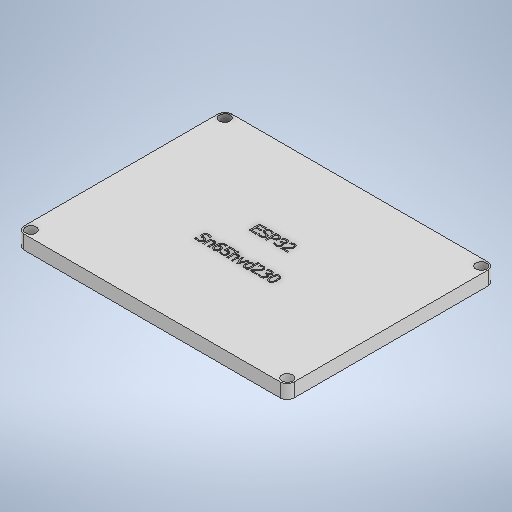
# Autodesk Inventor part: esp_can_case_lid
Saved by Autodesk Inventor 2025 (Build 290162000, 162)
## iProperties
Created: 2025-01-20
Part Number: esp_can_case_lid
Material: Generic
Document SubType Name: Modeling
Designer: danielrachi
Density: 1 g/cm^3
Appearance: Default
Author: danielrachi
Autodesk Inventor part; units mm, degrees
ref_plane "YZ Plane" through (0, 0, 0) normal (1, 0, 0) x (0, 1, 0)
ref_plane "XZ Plane" through (0, 0, 0) normal (0, 1, 0) x (-1, 0, 0)
ref_plane "XY Plane" through (0, 0, 0) normal (0, 0, 1) x (1, 0, 0)
sketch "Sketch1" plane through (0, 0, 0) normal (0, 1, 0) x (-1, 0, 0)
  line L0 (-39, 30) -> (39, 30)
  line L1 (39, 30) -> (39, -30)
  line L2 (39, -30) -> (-39, -30)
  line L3 (-39, -30) -> (-39, 30)
  line L4 (-39, 30) -> (39, -30) construction
  line L5 (39, 30) -> (-39, -30) construction
  point P0 (0, 0)
  dimension "d0" = 78
  dimension "d1" = 60
  constraints: 12 end point, 2 midpoint, 2 parallel, 1 horizontal, 1 perpendicular
  measures "d0" distance of L1.end L2.end
  measures "d1" distance of L0.end L1.end
extrude "Extrusion1" add sketch "Sketch1" along normal blind 4
sketch "Sketch2" plane through (0, 4, 0) normal (0, 1, 0) x (1, 0, 0)
  circle A0 centre (37, -28) radius 1.55
  line L0 (-39, -30) -> (39, -30) projected
  line L1 (39, -30) -> (39, 30) projected
  line L2 (-39, 30) -> (-39, -30) projected
  line L3 (-39, 0) -> (39, 0)
  line L4 (39, 30) -> (-39, 30) projected
  line L5 (0, 30) -> (0, -30)
  circle A1 centre (-37, -28) radius 1.55
  circle A2 centre (37, 28) radius 1.55
  circle A3 centre (-37, 28) radius 1.55
  line L6 (-39, 30) -> (39, 30) construction
  line L7 (39, 30) -> (39, -30) construction
  line L8 (39, -30) -> (-39, -30) construction
  line L9 (-39, -30) -> (-39, 30) construction
  line L10 (-5.4773, 3.4945) -> (-5.4773, 6.5425)
  line L11 (-5.4773, 6.5425) -> (-3.5704, 6.5425)
  line L12 (-3.5704, 6.5425) -> (-3.5704, 6.1818)
  line L13 (-3.5704, 6.1818) -> (-5.0722, 6.1818)
  line L14 (-5.0722, 6.1818) -> (-5.0722, 5.347)
  line L15 (-5.0722, 5.347) -> (-3.6717, 5.347)
  line L16 (-3.6717, 5.347) -> (-3.6717, 4.9863)
  line L17 (-3.6717, 4.9863) -> (-5.0722, 4.9863)
  line L18 (-5.0722, 4.9863) -> (-5.0722, 3.8551)
  line L19 (-5.0722, 3.8551) -> (-3.5704, 3.8551)
  line L20 (-3.5704, 3.8551) -> (-3.5704, 3.4945)
  line L21 (-3.5704, 3.4945) -> (-5.4773, 3.4945)
  spline S0 degree 2 poles (-2.2761, 3.4401) (-2.6071, 3.4401) (-3.0715, 3.5784) (-3.2765, 3.6772) knots 0 0 0 1 2 2 2
  line L22 (-3.2765, 3.6772) -> (-3.2765, 4.1861)
  line L23 (-3.2765, 4.1861) -> (-3.2468, 4.1861)
  spline S1 degree 2 poles (-3.2468, 4.1861) (-3.0468, 3.9983) (-2.5404, 3.7909) (-2.3058, 3.7909) knots 0 0 0 1 2 2 2
  spline S2 degree 2 poles (-2.3058, 3.7909) (-1.9698, 3.7909) (-1.6265, 4.07) (-1.6265, 4.2997) knots 0 0 0 1 2 2 2
  spline S3 degree 2 poles (-1.6265, 4.2997) (-1.6265, 4.4825) (-1.8068, 4.7097) (-2.0019, 4.7665) knots 0 0 0 1 2 2 2
  spline S4 degree 2 poles (-2.0019, 4.7665) (-2.1427, 4.806) (-2.3774, 4.8604) (-2.5528, 4.9048) knots 0 0 0 1 2 2 2
  spline S5 degree 2 poles (-2.5528, 4.9048) (-2.7108, 4.9468) (-2.9603, 5.0728) (-3.0566, 5.1741) knots 0 0 0 1 2 2 2
  spline S6 degree 2 poles (-3.0566, 5.1741) (-3.1505, 5.2753) (-3.2542, 5.547) (-3.2542, 5.7249) knots 0 0 0 1 2 2 2
  spline S7 degree 2 poles (-3.2542, 5.7249) (-3.2542, 6.0954) (-2.6763, 6.5968) (-2.2292, 6.5968) knots 0 0 0 1 2 2 2
  spline S8 degree 2 poles (-2.2292, 6.5968) (-1.9723, 6.5968) (-1.5178, 6.4955) (-1.3227, 6.3992) knots 0 0 0 1 2 2 2
  line L24 (-1.3227, 6.3992) -> (-1.3227, 5.9151)
  line L25 (-1.3227, 5.9151) -> (-1.3523, 5.9151)
  spline S9 degree 2 poles (-1.3523, 5.9151) (-1.4981, 6.0484) (-1.9525, 6.246) (-2.202, 6.246) knots 0 0 0 1 2 2 2
  spline S10 degree 2 poles (-2.202, 6.246) (-2.4836, 6.246) (-2.8319, 5.9818) (-2.8319, 5.7669) knots 0 0 0 1 2 2 2
  spline S11 degree 2 poles (-2.8319, 5.7669) (-2.8319, 5.5742) (-2.6269, 5.3445) (-2.4342, 5.2926) knots 0 0 0 1 2 2 2
  spline S12 degree 2 poles (-2.4342, 5.2926) (-2.3058, 5.258) (-1.9328, 5.1691) (-1.8093, 5.1321) knots 0 0 0 1 2 2 2
  spline S13 degree 2 poles (-1.8093, 5.1321) (-1.4956, 5.0357) (-1.2041, 4.6479) (-1.2041, 4.3639) knots 0 0 0 1 2 2 2
  spline S14 degree 2 poles (-1.2041, 4.3639) (-1.2041, 4.1836) (-1.3499, 3.8378) (-1.4808, 3.7168) knots 0 0 0 1 2 2 2
  spline S15 degree 2 poles (-1.4808, 3.7168) (-1.6265, 3.5834) (-1.997, 3.4401) (-2.2761, 3.4401) knots 0 0 0 1 2 2 2
  spline S16 degree 2 poles (1.135, 5.6236) (1.135, 5.426) (0.9942, 5.0703) (0.8682, 4.9468) knots 0 0 0 1 2 2 2
  spline S17 degree 2 poles (0.8682, 4.9468) (0.7101, 4.7912) (0.2828, 4.6307) (-0.0432, 4.6307) knots 0 0 0 1 2 2 2
  line L26 (-0.0432, 4.6307) -> (-0.3866, 4.6307)
  line L27 (-0.3866, 4.6307) -> (-0.3866, 3.4945)
  line L28 (-0.3866, 3.4945) -> (-0.7916, 3.4945)
  line L29 (-0.7916, 3.4945) -> (-0.7916, 6.5425)
  line L30 (-0.7916, 6.5425) -> (-0.0259, 6.5425)
  spline S18 degree 2 poles (-0.0259, 6.5425) (0.2458, 6.5425) (0.6261, 6.4535) (0.7719, 6.3523) knots 0 0 0 1 2 2 2
  spline S19 degree 2 poles (0.7719, 6.3523) (0.9423, 6.2362) (1.135, 5.878) (1.135, 5.6236) knots 0 0 0 1 2 2 2
  spline S20 degree 2 poles (0.7126, 5.6113) (0.7126, 5.7693) (0.6039, 6.0015) (0.4928, 6.0756) knots 0 0 0 1 2 2 2
  spline S21 degree 2 poles (0.4928, 6.0756) (0.3964, 6.1398) (0.1396, 6.1917) (-0.0506, 6.1917) knots 0 0 0 1 2 2 2
  line L31 (-0.0506, 6.1917) -> (-0.3866, 6.1917)
  line L32 (-0.3866, 6.1917) -> (-0.3866, 4.9765)
  line L33 (-0.3866, 4.9765) -> (-0.1099, 4.9765)
  spline S22 degree 2 poles (-0.1099, 4.9765) (0.1371, 4.9765) (0.4409, 5.0555) (0.5397, 5.1592) knots 0 0 0 1 2 2 2
  spline S23 degree 2 poles (0.5397, 5.1592) (0.6311, 5.2506) (0.7126, 5.4655) (0.7126, 5.6113) knots 0 0 0 1 2 2 2
  spline S24 degree 2 poles (2.2564, 6.2535) (2.1452, 6.2535) (1.9254, 6.1991) (1.8192, 6.1571) knots 0 0 0 1 2 2 2
  spline S25 degree 2 poles (1.8192, 6.1571) (1.7204, 6.1151) (1.5746, 6.0262) (1.5178, 5.9867) knots 0 0 0 1 2 2 2
  line L34 (1.5178, 5.9867) -> (1.4931, 5.9867)
  line L35 (1.4931, 5.9867) -> (1.4931, 6.419)
  spline S26 degree 2 poles (1.4931, 6.419) (1.6265, 6.4906) (2.0835, 6.6067) (2.2885, 6.6067) knots 0 0 0 1 2 2 2
  spline S27 degree 2 poles (2.2885, 6.6067) (2.496, 6.6067) (2.8047, 6.5227) (2.9307, 6.4338) knots 0 0 0 1 2 2 2
  spline S28 degree 2 poles (2.9307, 6.4338) (3.0641, 6.3374) (3.2024, 6.0583) (3.2024, 5.8706) knots 0 0 0 1 2 2 2
  spline S29 degree 2 poles (3.2024, 5.8706) (3.2024, 5.6187) (2.8714, 5.2383) (2.6392, 5.1889) knots 0 0 0 1 2 2 2
  line L36 (2.6392, 5.1889) -> (2.6392, 5.1592)
  spline S30 degree 2 poles (2.6392, 5.1592) (2.7355, 5.1395) (2.9554, 5.0506) (3.0492, 4.9616) knots 0 0 0 1 2 2 2
  spline S31 degree 2 poles (3.0492, 4.9616) (3.1431, 4.8752) (3.2617, 4.5985) (3.2617, 4.3985) knots 0 0 0 1 2 2 2
  spline S32 degree 2 poles (3.2617, 4.3985) (3.2617, 4.1935) (3.1209, 3.8452) (2.9924, 3.7118) knots 0 0 0 1 2 2 2
  spline S33 degree 2 poles (2.9924, 3.7118) (2.859, 3.5735) (2.4811, 3.4302) (2.2415, 3.4302) knots 0 0 0 1 2 2 2
  spline S34 degree 2 poles (2.2415, 3.4302) (2.0118, 3.4302) (1.5623, 3.5414) (1.4091, 3.618) knots 0 0 0 1 2 2 2
  line L37 (1.4091, 3.618) -> (1.4091, 4.0502)
  line L38 (1.4091, 4.0502) -> (1.4388, 4.0502)
  spline S35 degree 2 poles (1.4388, 4.0502) (1.5672, 3.9563) (2.0019, 3.7834) (2.2168, 3.7834) knots 0 0 0 1 2 2 2
  spline S36 degree 2 poles (2.2168, 3.7834) (2.3428, 3.7834) (2.5948, 3.8625) (2.6787, 3.9539) knots 0 0 0 1 2 2 2
  spline S37 degree 2 poles (2.6787, 3.9539) (2.7602, 4.0453) (2.8467, 4.2626) (2.8467, 4.4281) knots 0 0 0 1 2 2 2
  spline S38 degree 2 poles (2.8467, 4.4281) (2.8467, 4.5936) (2.7504, 4.8085) (2.6639, 4.8703) knots 0 0 0 1 2 2 2
  spline S39 degree 2 poles (2.6639, 4.8703) (2.5775, 4.932) (2.3428, 4.9789) (2.2045, 4.9789) knots 0 0 0 1 2 2 2
  line L39 (2.2045, 4.9789) -> (2.0316, 4.9789)
  line L40 (2.0316, 4.9789) -> (2.0316, 5.3173)
  line L41 (2.0316, 5.3173) -> (2.1674, 5.3173)
  spline S40 degree 2 poles (2.1674, 5.3173) (2.4416, 5.3173) (2.7874, 5.5791) (2.7874, 5.8286) knots 0 0 0 1 2 2 2
  spline S41 degree 2 poles (2.7874, 5.8286) (2.7874, 5.9447) (2.6985, 6.1102) (2.6269, 6.1596) knots 0 0 0 1 2 2 2
  spline S42 degree 2 poles (2.6269, 6.1596) (2.5503, 6.2115) (2.3626, 6.2535) (2.2564, 6.2535) knots 0 0 0 1 2 2 2
  line L42 (5.6008, 3.4945) -> (3.7211, 3.4945)
  line L43 (3.7211, 3.4945) -> (3.7211, 3.9267)
  spline S43 degree 2 poles (3.7211, 3.9267) (3.9236, 4.1169) (4.2842, 4.4701) (4.4571, 4.6603) knots 0 0 0 1 2 2 2
  spline S44 degree 2 poles (4.4571, 4.6603) (4.8054, 5.0432) (5.0598, 5.5026) (5.0598, 5.7471) knots 0 0 0 1 2 2 2
  spline S45 degree 2 poles (5.0598, 5.7471) (5.0598, 5.8755) (4.9808, 6.0682) (4.9092, 6.13) knots 0 0 0 1 2 2 2
  spline S46 degree 2 poles (4.9092, 6.13) (4.8375, 6.1917) (4.6498, 6.2535) (4.5362, 6.2535) knots 0 0 0 1 2 2 2
  spline S47 degree 2 poles (4.5362, 6.2535) (4.4275, 6.2535) (4.2052, 6.1991) (4.1039, 6.1571) knots 0 0 0 1 2 2 2
  spline S48 degree 2 poles (4.1039, 6.1571) (4.0175, 6.1225) (3.8569, 6.0237) (3.8075, 5.9892) knots 0 0 0 1 2 2 2
  line L44 (3.8075, 5.9892) -> (3.7853, 5.9892)
  line L45 (3.7853, 5.9892) -> (3.7853, 6.4239)
  spline S49 degree 2 poles (3.7853, 6.4239) (3.9113, 6.4856) (4.3633, 6.6067) (4.5658, 6.6067) knots 0 0 0 1 2 2 2
  spline S50 degree 2 poles (4.5658, 6.6067) (4.9931, 6.6067) (5.4748, 6.1547) (5.4748, 5.7693) knots 0 0 0 1 2 2 2
  spline S51 degree 2 poles (5.4748, 5.7693) (5.4748, 5.589) (5.3908, 5.2877) (5.3167, 5.1592) knots 0 0 0 1 2 2 2
  spline S52 degree 2 poles (5.3167, 5.1592) (5.2426, 5.0259) (5.0277, 4.764) (4.9092, 4.6381) knots 0 0 0 1 2 2 2
  spline S53 degree 2 poles (4.9092, 4.6381) (4.7165, 4.4281) (4.2447, 3.9786) (4.1039, 3.8477) knots 0 0 0 1 2 2 2
  line L46 (4.1039, 3.8477) -> (5.6008, 3.8477)
  line L47 (5.6008, 3.8477) -> (5.6008, 3.4945)
  spline S54 degree 2 poles (-10.2654, -6.5968) (-10.5964, -6.5968) (-11.0607, -6.4585) (-11.2657, -6.3597) knots 0 0 0 1 2 2 2
  line L48 (-11.2657, -6.3597) -> (-11.2657, -5.8508)
  line L49 (-11.2657, -5.8508) -> (-11.2361, -5.8508)
  spline S55 degree 2 poles (-11.2361, -5.8508) (-11.036, -6.0386) (-10.5297, -6.246) (-10.295, -6.246) knots 0 0 0 1 2 2 2
  spline S56 degree 2 poles (-10.295, -6.246) (-9.9591, -6.246) (-9.6158, -5.9669) (-9.6158, -5.7372) knots 0 0 0 1 2 2 2
  spline S57 degree 2 poles (-9.6158, -5.7372) (-9.6158, -5.5544) (-9.7961, -5.3272) (-9.9912, -5.2704) knots 0 0 0 1 2 2 2
  spline S58 degree 2 poles (-9.9912, -5.2704) (-10.132, -5.2309) (-10.3667, -5.1765) (-10.542, -5.1321) knots 0 0 0 1 2 2 2
  spline S59 degree 2 poles (-10.542, -5.1321) (-10.7001, -5.0901) (-10.9496, -4.9641) (-11.0459, -4.8628) knots 0 0 0 1 2 2 2
  spline S60 degree 2 poles (-11.0459, -4.8628) (-11.1398, -4.7616) (-11.2435, -4.4899) (-11.2435, -4.312) knots 0 0 0 1 2 2 2
  spline S61 degree 2 poles (-11.2435, -4.312) (-11.2435, -3.9415) (-10.6655, -3.4401) (-10.2185, -3.4401) knots 0 0 0 1 2 2 2
  spline S62 degree 2 poles (-10.2185, -3.4401) (-9.9616, -3.4401) (-9.5071, -3.5414) (-9.312, -3.6377) knots 0 0 0 1 2 2 2
  line L50 (-9.312, -3.6377) -> (-9.312, -4.1218)
  line L51 (-9.312, -4.1218) -> (-9.3416, -4.1218)
  spline S63 degree 2 poles (-9.3416, -4.1218) (-9.4873, -3.9885) (-9.9418, -3.7909) (-10.1913, -3.7909) knots 0 0 0 1 2 2 2
  spline S64 degree 2 poles (-10.1913, -3.7909) (-10.4729, -3.7909) (-10.8211, -4.0551) (-10.8211, -4.27) knots 0 0 0 1 2 2 2
  spline S65 degree 2 poles (-10.8211, -4.27) (-10.8211, -4.4627) (-10.6161, -4.6924) (-10.4235, -4.7443) knots 0 0 0 1 2 2 2
  spline S66 degree 2 poles (-10.4235, -4.7443) (-10.295, -4.7789) (-9.9221, -4.8678) (-9.7986, -4.9048) knots 0 0 0 1 2 2 2
  spline S67 degree 2 poles (-9.7986, -4.9048) (-9.4849, -5.0012) (-9.1934, -5.389) (-9.1934, -5.673) knots 0 0 0 1 2 2 2
  spline S68 degree 2 poles (-9.1934, -5.673) (-9.1934, -5.8533) (-9.3391, -6.1991) (-9.47, -6.3202) knots 0 0 0 1 2 2 2
  spline S69 degree 2 poles (-9.47, -6.3202) (-9.6158, -6.4535) (-9.9863, -6.5968) (-10.2654, -6.5968) knots 0 0 0 1 2 2 2
  line L52 (-7.0148, -6.5425) -> (-7.4002, -6.5425)
  line L53 (-7.4002, -6.5425) -> (-7.4002, -5.2383)
  spline S70 degree 2 poles (-7.4002, -5.2383) (-7.4002, -5.0802) (-7.4298, -4.8085) (-7.4743, -4.727) knots 0 0 0 1 2 2 2
  spline S71 degree 2 poles (-7.4743, -4.727) (-7.5212, -4.6405) (-7.6892, -4.5566) (-7.8324, -4.5566) knots 0 0 0 1 2 2 2
  spline S72 degree 2 poles (-7.8324, -4.5566) (-7.9757, -4.5566) (-8.2795, -4.7097) (-8.4252, -4.8332) knots 0 0 0 1 2 2 2
  line L54 (-8.4252, -4.8332) -> (-8.4252, -6.5425)
  line L55 (-8.4252, -6.5425) -> (-8.8105, -6.5425)
  line L56 (-8.8105, -6.5425) -> (-8.8105, -4.2552)
  line L57 (-8.8105, -4.2552) -> (-8.4252, -4.2552)
  line L58 (-8.4252, -4.2552) -> (-8.4252, -4.5096)
  spline S73 degree 2 poles (-8.4252, -4.5096) (-8.2523, -4.354) (-7.9189, -4.191) (-7.7312, -4.191) knots 0 0 0 1 2 2 2
  spline S74 degree 2 poles (-7.7312, -4.191) (-7.3952, -4.191) (-7.0148, -4.6356) (-7.0148, -5.058) knots 0 0 0 1 2 2 2
  line L59 (-7.0148, -5.058) -> (-7.0148, -6.5425)
  spline S75 degree 2 poles (-4.6041, -5.5544) (-4.6041, -5.7891) (-4.7597, -6.1868) (-4.8906, -6.3202) knots 0 0 0 1 2 2 2
  spline S76 degree 2 poles (-4.8906, -6.3202) (-5.0265, -6.4609) (-5.3673, -6.6067) (-5.5724, -6.6067) knots 0 0 0 1 2 2 2
  spline S77 degree 2 poles (-5.5724, -6.6067) (-5.7774, -6.6067) (-6.1158, -6.4684) (-6.2442, -6.33) knots 0 0 0 1 2 2 2
  spline S78 degree 2 poles (-6.2442, -6.33) (-6.4023, -6.1645) (-6.5801, -5.6088) (-6.5801, -5.2037) knots 0 0 0 1 2 2 2
  spline S79 degree 2 poles (-6.5801, -5.2037) (-6.5801, -4.806) (-6.4171, -4.1663) (-6.2467, -3.9292) knots 0 0 0 1 2 2 2
  spline S80 degree 2 poles (-6.2467, -3.9292) (-6.0812, -3.697) (-5.5575, -3.4376) (-5.2142, -3.4376) knots 0 0 0 1 2 2 2
  spline S81 degree 2 poles (-5.2142, -3.4376) (-5.1129, -3.4376) (-4.9351, -3.4574) (-4.8684, -3.4796) knots 0 0 0 1 2 2 2
  line L60 (-4.8684, -3.4796) -> (-4.8684, -3.8724)
  line L61 (-4.8684, -3.8724) -> (-4.8857, -3.8724)
  spline S82 degree 2 poles (-4.8857, -3.8724) (-4.9425, -3.8427) (-5.15, -3.7909) (-5.2685, -3.7909) knots 0 0 0 1 2 2 2
  spline S83 degree 2 poles (-5.2685, -3.7909) (-5.6489, -3.7909) (-6.1158, -4.3046) (-6.1602, -4.8085) knots 0 0 0 1 2 2 2
  spline S84 degree 2 poles (-6.1602, -4.8085) (-6.0145, -4.7072) (-5.7082, -4.5961) (-5.5254, -4.5961) knots 0 0 0 1 2 2 2
  spline S85 degree 2 poles (-5.5254, -4.5961) (-5.3476, -4.5961) (-5.0808, -4.6677) (-4.9351, -4.7764) knots 0 0 0 1 2 2 2
  spline S86 degree 2 poles (-4.9351, -4.7764) (-4.7671, -4.9024) (-4.6041, -5.2926) (-4.6041, -5.5544) knots 0 0 0 1 2 2 2
  spline S87 degree 2 poles (-5.0191, -5.5717) (-5.0191, -5.384) (-5.1179, -5.1296) (-5.2266, -5.0407) knots 0 0 0 1 2 2 2
  spline S88 degree 2 poles (-5.2266, -5.0407) (-5.3081, -4.9765) (-5.5106, -4.9345) (-5.6168, -4.9345) knots 0 0 0 1 2 2 2
  spline S89 degree 2 poles (-5.6168, -4.9345) (-5.7601, -4.9345) (-6.0293, -5.0209) (-6.1602, -5.1024) knots 0 0 0 1 2 2 2
  spline S90 degree 2 poles (-6.1602, -5.1024) (-6.1627, -5.1469) (-6.1676, -5.2309) (-6.1676, -5.2951) knots 0 0 0 1 2 2 2
  spline S91 degree 2 poles (-6.1676, -5.2951) (-6.1676, -5.6113) (-6.0441, -5.999) (-5.9503, -6.1003) knots 0 0 0 1 2 2 2
  spline S92 degree 2 poles (-5.9503, -6.1003) (-5.8638, -6.1966) (-5.6761, -6.2732) (-5.5699, -6.2732) knots 0 0 0 1 2 2 2
  spline S93 degree 2 poles (-5.5699, -6.2732) (-5.3229, -6.2732) (-5.0191, -5.9225) (-5.0191, -5.5717) knots 0 0 0 1 2 2 2
  spline S94 degree 2 poles (-2.3959, -5.5742) (-2.3959, -5.794) (-2.5367, -6.1695) (-2.6651, -6.3078) knots 0 0 0 1 2 2 2
  spline S95 degree 2 poles (-2.6651, -6.3078) (-2.7936, -6.4461) (-3.1764, -6.6067) (-3.4136, -6.6067) knots 0 0 0 1 2 2 2
  spline S96 degree 2 poles (-3.4136, -6.6067) (-3.6309, -6.6067) (-4.0558, -6.5103) (-4.2114, -6.4338) knots 0 0 0 1 2 2 2
  line L62 (-4.2114, -6.4338) -> (-4.2114, -6.0015)
  line L63 (-4.2114, -6.0015) -> (-4.1817, -6.0015)
  spline S97 degree 2 poles (-4.1817, -6.0015) (-4.1348, -6.0361) (-3.9594, -6.125) (-3.8532, -6.1645) knots 0 0 0 1 2 2 2
  spline S98 degree 2 poles (-3.8532, -6.1645) (-3.7322, -6.2065) (-3.5321, -6.2535) (-3.4062, -6.2535) knots 0 0 0 1 2 2 2
  spline S99 degree 2 poles (-3.4062, -6.2535) (-3.2827, -6.2535) (-3.0505, -6.1645) (-2.9665, -6.0682) knots 0 0 0 1 2 2 2
  spline S100 degree 2 poles (-2.9665, -6.0682) (-2.8899, -5.9768) (-2.8109, -5.7348) (-2.8109, -5.5717) knots 0 0 0 1 2 2 2
  spline S101 degree 2 poles (-2.8109, -5.5717) (-2.8109, -5.4087) (-2.8998, -5.2012) (-2.9838, -5.1321) knots 0 0 0 1 2 2 2
  spline S102 degree 2 poles (-2.9838, -5.1321) (-3.0702, -5.0555) (-3.3271, -4.9913) (-3.4827, -4.9913) knots 0 0 0 1 2 2 2
  spline S103 degree 2 poles (-3.4827, -4.9913) (-3.6507, -4.9913) (-3.9841, -5.0432) (-4.0854, -5.0654) knots 0 0 0 1 2 2 2
  line L64 (-4.0854, -5.0654) -> (-4.0854, -3.4945)
  line L65 (-4.0854, -3.4945) -> (-2.4132, -3.4945)
  line L66 (-2.4132, -3.4945) -> (-2.4132, -3.8526)
  line L67 (-2.4132, -3.8526) -> (-3.6927, -3.8526)
  line L68 (-3.6927, -3.8526) -> (-3.6927, -4.6652)
  spline S104 degree 2 poles (-3.6927, -4.6652) (-3.6186, -4.6554) (-3.4753, -4.6479) (-3.416, -4.6479) knots 0 0 0 1 2 2 2
  spline S105 degree 2 poles (-3.416, -4.6479) (-3.1814, -4.6479) (-2.8578, -4.7245) (-2.7096, -4.8381) knots 0 0 0 1 2 2 2
  spline S106 degree 2 poles (-2.7096, -4.8381) (-2.5589, -4.9518) (-2.3959, -5.2976) (-2.3959, -5.5742) knots 0 0 0 1 2 2 2
  line L69 (-0.1037, -6.5425) -> (-0.4891, -6.5425)
  line L70 (-0.4891, -6.5425) -> (-0.4891, -5.2383)
  spline S107 degree 2 poles (-0.4891, -5.2383) (-0.4891, -5.0802) (-0.5187, -4.8085) (-0.5632, -4.727) knots 0 0 0 1 2 2 2
  spline S108 degree 2 poles (-0.5632, -4.727) (-0.6101, -4.6405) (-0.7781, -4.5566) (-0.9213, -4.5566) knots 0 0 0 1 2 2 2
  spline S109 degree 2 poles (-0.9213, -4.5566) (-1.0646, -4.5566) (-1.3684, -4.7097) (-1.5141, -4.8332) knots 0 0 0 1 2 2 2
  line L71 (-1.5141, -4.8332) -> (-1.5141, -6.5425)
  line L72 (-1.5141, -6.5425) -> (-1.8994, -6.5425)
  line L73 (-1.8994, -6.5425) -> (-1.8994, -3.3586)
  line L74 (-1.8994, -3.3586) -> (-1.5141, -3.3586)
  line L75 (-1.5141, -3.3586) -> (-1.5141, -4.5096)
  spline S110 degree 2 poles (-1.5141, -4.5096) (-1.3412, -4.354) (-1.0078, -4.191) (-0.82, -4.191) knots 0 0 0 1 2 2 2
  spline S111 degree 2 poles (-0.82, -4.191) (-0.4841, -4.191) (-0.1037, -4.6356) (-0.1037, -5.058) knots 0 0 0 1 2 2 2
  line L76 (-0.1037, -5.058) -> (-0.1037, -6.5425)
  line L77 (2.2329, -4.2552) -> (1.3709, -6.5425)
  line L78 (1.3709, -6.5425) -> (1.0251, -6.5425)
  line L79 (1.0251, -6.5425) -> (0.1704, -4.2552)
  line L80 (0.1704, -4.2552) -> (0.5879, -4.2552)
  line L81 (0.5879, -4.2552) -> (1.2128, -6.0163)
  line L82 (1.2128, -6.0163) -> (1.8328, -4.2552)
  line L83 (1.8328, -4.2552) -> (2.2329, -4.2552)
  line L84 (4.283, -6.5425) -> (3.8977, -6.5425)
  line L85 (3.8977, -6.5425) -> (3.8977, -6.3103)
  spline S112 degree 2 poles (3.8977, -6.3103) (3.8088, -6.3844) (3.6779, -6.4832) (3.5889, -6.5252) knots 0 0 0 1 2 2 2
  spline S113 degree 2 poles (3.5889, -6.5252) (3.5074, -6.5647) (3.3321, -6.6067) (3.216, -6.6067) knots 0 0 0 1 2 2 2
  spline S114 degree 2 poles (3.216, -6.6067) (3.0282, -6.6067) (2.7121, -6.4511) (2.6009, -6.3004) knots 0 0 0 1 2 2 2
  spline S115 degree 2 poles (2.6009, -6.3004) (2.4898, -6.1497) (2.3663, -5.7051) (2.3663, -5.4161) knots 0 0 0 1 2 2 2
  spline S116 degree 2 poles (2.3663, -5.4161) (2.3663, -5.1148) (2.5219, -4.6751) (2.6577, -4.5096) knots 0 0 0 1 2 2 2
  spline S117 degree 2 poles (2.6577, -4.5096) (2.7837, -4.3614) (3.1369, -4.191) (3.3321, -4.191) knots 0 0 0 1 2 2 2
  spline S118 degree 2 poles (3.3321, -4.191) (3.5025, -4.191) (3.7569, -4.2676) (3.8977, -4.3466) knots 0 0 0 1 2 2 2
  line L86 (3.8977, -4.3466) -> (3.8977, -3.3586)
  line L87 (3.8977, -3.3586) -> (4.283, -3.3586)
  line L88 (4.283, -3.3586) -> (4.283, -6.5425)
  line L89 (3.8977, -5.9867) -> (3.8977, -4.6652)
  spline S119 degree 2 poles (3.8977, -4.6652) (3.7544, -4.5961) (3.5272, -4.5442) (3.3963, -4.5442) knots 0 0 0 1 2 2 2
  spline S120 degree 2 poles (3.3963, -4.5442) (3.0999, -4.5442) (2.7639, -4.9888) (2.7639, -5.4087) knots 0 0 0 1 2 2 2
  spline S121 degree 2 poles (2.7639, -5.4087) (2.7639, -5.8138) (3.0208, -6.2411) (3.3049, -6.2411) knots 0 0 0 1 2 2 2
  spline S122 degree 2 poles (3.3049, -6.2411) (3.4556, -6.2411) (3.7618, -6.1028) (3.8977, -5.9867) knots 0 0 0 1 2 2 2
  line L90 (6.6641, -6.5425) -> (4.7844, -6.5425)
  line L91 (4.7844, -6.5425) -> (4.7844, -6.1102)
  spline S123 degree 2 poles (4.7844, -6.1102) (4.987, -5.92) (5.3476, -5.5668) (5.5205, -5.3766) knots 0 0 0 1 2 2 2
  spline S124 degree 2 poles (5.5205, -5.3766) (5.8688, -4.9938) (6.1232, -4.5343) (6.1232, -4.2898) knots 0 0 0 1 2 2 2
  spline S125 degree 2 poles (6.1232, -4.2898) (6.1232, -4.1614) (6.0441, -3.9687) (5.9725, -3.9069) knots 0 0 0 1 2 2 2
  spline S126 degree 2 poles (5.9725, -3.9069) (5.9009, -3.8452) (5.7131, -3.7834) (5.5995, -3.7834) knots 0 0 0 1 2 2 2
  spline S127 degree 2 poles (5.5995, -3.7834) (5.4908, -3.7834) (5.2685, -3.8378) (5.1673, -3.8798) knots 0 0 0 1 2 2 2
  spline S128 degree 2 poles (5.1673, -3.8798) (5.0808, -3.9144) (4.9203, -4.0132) (4.8709, -4.0477) knots 0 0 0 1 2 2 2
  line L92 (4.8709, -4.0477) -> (4.8486, -4.0477)
  line L93 (4.8486, -4.0477) -> (4.8486, -3.613)
  spline S129 degree 2 poles (4.8486, -3.613) (4.9746, -3.5513) (5.4266, -3.4302) (5.6292, -3.4302) knots 0 0 0 1 2 2 2
  spline S130 degree 2 poles (5.6292, -3.4302) (6.0565, -3.4302) (6.5381, -3.8822) (6.5381, -4.2676) knots 0 0 0 1 2 2 2
  spline S131 degree 2 poles (6.5381, -4.2676) (6.5381, -4.4479) (6.4542, -4.7492) (6.3801, -4.8777) knots 0 0 0 1 2 2 2
  spline S132 degree 2 poles (6.3801, -4.8777) (6.306, -5.011) (6.0911, -5.2729) (5.9725, -5.3988) knots 0 0 0 1 2 2 2
  spline S133 degree 2 poles (5.9725, -5.3988) (5.7798, -5.6088) (5.3081, -6.0583) (5.1673, -6.1892) knots 0 0 0 1 2 2 2
  line L94 (5.1673, -6.1892) -> (6.6641, -6.1892)
  line L95 (6.6641, -6.1892) -> (6.6641, -6.5425)
  spline S134 degree 2 poles (7.8942, -3.7834) (7.783, -3.7834) (7.5632, -3.8378) (7.457, -3.8798) knots 0 0 0 1 2 2 2
  spline S135 degree 2 poles (7.457, -3.8798) (7.3582, -3.9218) (7.2124, -4.0107) (7.1556, -4.0502) knots 0 0 0 1 2 2 2
  line L96 (7.1556, -4.0502) -> (7.1309, -4.0502)
  line L97 (7.1309, -4.0502) -> (7.1309, -3.618)
  spline S136 degree 2 poles (7.1309, -3.618) (7.2643, -3.5463) (7.7213, -3.4302) (7.9263, -3.4302) knots 0 0 0 1 2 2 2
  spline S137 degree 2 poles (7.9263, -3.4302) (8.1338, -3.4302) (8.4425, -3.5142) (8.5685, -3.6031) knots 0 0 0 1 2 2 2
  spline S138 degree 2 poles (8.5685, -3.6031) (8.7019, -3.6995) (8.8402, -3.9786) (8.8402, -4.1663) knots 0 0 0 1 2 2 2
  spline S139 degree 2 poles (8.8402, -4.1663) (8.8402, -4.4182) (8.5092, -4.7986) (8.277, -4.848) knots 0 0 0 1 2 2 2
  line L98 (8.277, -4.848) -> (8.277, -4.8777)
  spline S140 degree 2 poles (8.277, -4.8777) (8.3734, -4.8974) (8.5932, -4.9863) (8.687, -5.0753) knots 0 0 0 1 2 2 2
  spline S141 degree 2 poles (8.687, -5.0753) (8.7809, -5.1617) (8.8995, -5.4384) (8.8995, -5.6384) knots 0 0 0 1 2 2 2
  spline S142 degree 2 poles (8.8995, -5.6384) (8.8995, -5.8434) (8.7587, -6.1917) (8.6302, -6.3251) knots 0 0 0 1 2 2 2
  spline S143 degree 2 poles (8.6302, -6.3251) (8.4969, -6.4634) (8.1189, -6.6067) (7.8794, -6.6067) knots 0 0 0 1 2 2 2
  spline S144 degree 2 poles (7.8794, -6.6067) (7.6496, -6.6067) (7.2001, -6.4955) (7.047, -6.419) knots 0 0 0 1 2 2 2
  line L99 (7.047, -6.419) -> (7.047, -5.9867)
  line L100 (7.047, -5.9867) -> (7.0766, -5.9867)
  spline S145 degree 2 poles (7.0766, -5.9867) (7.205, -6.0806) (7.6398, -6.2535) (7.8547, -6.2535) knots 0 0 0 1 2 2 2
  spline S146 degree 2 poles (7.8547, -6.2535) (7.9806, -6.2535) (8.2326, -6.1744) (8.3165, -6.083) knots 0 0 0 1 2 2 2
  spline S147 degree 2 poles (8.3165, -6.083) (8.3981, -5.9916) (8.4845, -5.7743) (8.4845, -5.6088) knots 0 0 0 1 2 2 2
  spline S148 degree 2 poles (8.4845, -5.6088) (8.4845, -5.4433) (8.3882, -5.2284) (8.3017, -5.1667) knots 0 0 0 1 2 2 2
  spline S149 degree 2 poles (8.3017, -5.1667) (8.2153, -5.1049) (7.9806, -5.058) (7.8423, -5.058) knots 0 0 0 1 2 2 2
  line L101 (7.8423, -5.058) -> (7.6694, -5.058)
  line L102 (7.6694, -5.058) -> (7.6694, -4.7196)
  line L103 (7.6694, -4.7196) -> (7.8053, -4.7196)
  spline S150 degree 2 poles (7.8053, -4.7196) (8.0794, -4.7196) (8.4252, -4.4578) (8.4252, -4.2083) knots 0 0 0 1 2 2 2
  spline S151 degree 2 poles (8.4252, -4.2083) (8.4252, -4.0922) (8.3363, -3.9267) (8.2647, -3.8773) knots 0 0 0 1 2 2 2
  spline S152 degree 2 poles (8.2647, -3.8773) (8.1881, -3.8254) (8.0004, -3.7834) (7.8942, -3.7834) knots 0 0 0 1 2 2 2
  spline S153 degree 2 poles (11.2559, -5.0185) (11.2559, -5.8385) (10.7792, -6.6067) (10.2827, -6.6067) knots 0 0 0 1 2 2 2
  spline S154 degree 2 poles (10.2827, -6.6067) (9.7788, -6.6067) (9.307, -5.8237) (9.307, -5.0209) knots 0 0 0 1 2 2 2
  spline S155 degree 2 poles (9.307, -5.0209) (9.307, -4.1959) (9.7837, -3.4327) (10.2827, -3.4327) knots 0 0 0 1 2 2 2
  spline S156 degree 2 poles (10.2827, -3.4327) (10.7841, -3.4327) (11.2559, -4.2231) (11.2559, -5.0185) knots 0 0 0 1 2 2 2
  spline S157 degree 2 poles (10.7322, -5.9472) (10.7915, -5.7965) (10.8409, -5.3321) (10.8409, -5.0185) knots 0 0 0 1 2 2 2
  spline S158 degree 2 poles (10.8409, -5.0185) (10.8409, -4.7048) (10.7915, -4.2429) (10.7298, -4.0873) knots 0 0 0 1 2 2 2
  spline S159 degree 2 poles (10.7298, -4.0873) (10.668, -3.9316) (10.4531, -3.7711) (10.2827, -3.7711) knots 0 0 0 1 2 2 2
  spline S160 degree 2 poles (10.2827, -3.7711) (10.1122, -3.7711) (9.8924, -3.9316) (9.8282, -4.0922) knots 0 0 0 1 2 2 2
  spline S161 degree 2 poles (9.8282, -4.0922) (9.7664, -4.2478) (9.722, -4.722) (9.722, -5.0209) knots 0 0 0 1 2 2 2
  spline S162 degree 2 poles (9.722, -5.0209) (9.722, -5.342) (9.7615, -5.7718) (9.8257, -5.9398) knots 0 0 0 1 2 2 2
  spline S163 degree 2 poles (9.8257, -5.9398) (9.885, -6.0978) (10.1048, -6.2683) (10.2827, -6.2683) knots 0 0 0 1 2 2 2
  spline S164 degree 2 poles (10.2827, -6.2683) (10.4506, -6.2683) (10.6705, -6.1077) (10.7322, -5.9472) knots 0 0 0 1 2 2 2
  point P0 (0, 0)
  dimension "d4" = 3.1
  dimension "d5" = 2
  dimension "d6" = 2
  constraints: 4 centre point, 4 collinear, 4 end point, 4 midpoint, 3 symmetric about line, 5 other
  measures "d4" diameter of A0
  measures "d5" distance from line of A0.centre L0
  measures "d6" distance from line of A0.centre L1
extrude "Extrusion2" cut sketch "Sketch2" against normal blind 4 contours A0 | S17 L26 L27 L28 L29 L30 S18 L5 S21 L31 L32 L33 S22 | L5 S22 S23 S20 S21 S18 S19 S16 S17 | A1 | A2 | A3 | L10 L11 L12 L13 L14 L15 L16 L17 L18 L19 L20 L21 | S0 L22 L23 S1 S2 S3 S4 S5 S6 S7 S8 L24 L25 S9 S10 S11 S12 S13 S14 S15 | S24 S25 L34 L35 S26 S27 S28 S29 L36 S30 S31 S32 S33 S34 L37 L38 S35 S36 S37 S38 S39 L39 L40 L41 S40 S41 S42 | L42 L43 S43 S44 S45 S46 S47 S48 L44 L45 S49 S50 S51 S52 S53 L46 L47 | S54 L48 L49 S55 S56 S57 S58 S59 S60 S61 S62 L50 L51 S63 S64 S65 S66 S67 S68 S69 | L52 L53 S70 S71 S72 L54 L55 L56 L57 L58 S73 S74 L59 | S75 S76 S77 S78 S79 S80 S81 L60 L61 S82 S83 S84 S85 S86 | S94 S95 S96 L62 L63 S97 S98 S99 S100 S101 S102 S103 L64 L65 L66 L67 L68 S104 S105 S106 | L69 L70 S107 S108 S109 L71 L72 L73 L74 L75 S110 S111 L76 | L77 L78 L79 L80 L81 L82 L83 | L84 L85 S112 S113 S114 S115 S116 S117 S118 L86 L87 L88 | L90 L91 S123 S124 S125 S126 S127 S128 L92 L93 S129 S130 S131 S132 S133 L94 L95 | S134 S135 L96 L97 S136 S137 S138 S139 L98 S140 S141 S142 S143 S144 L99 L100 S145 S146 S147 S148 S149 L101 L102 L103 S150 S151 S152 | S153 S154 S155 S156
fillet "Fillet1" radius 2 4 edges at (-39, 2, 30) (39, 2, 30) (39, 2, -30) (-39, 2, -30)
body "Solid1"
